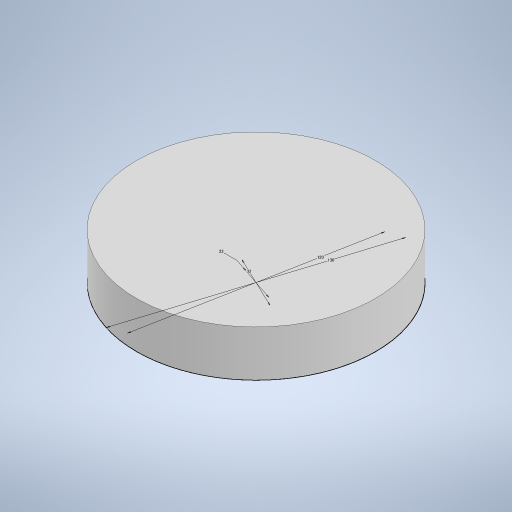
# Autodesk Inventor part: 18-1
Saved by Autodesk Inventor 2023 (Build 270158000, 158)
## iProperties
Created: 2022-11-18
Part Number: 18-1
Material: 一般
Document SubType Name: Modeling
Designer: RM206user
Density: 1 g/cm^3
Appearance: 既定
Author: RM206user
Autodesk Inventor part; units mm, degrees
ref_plane "YZ Plane" through (0, 0, 0) normal (1, 0, 0) x (0, 1, 0)
ref_plane "XZ Plane" through (0, 0, 0) normal (0, 1, 0) x (-1, 0, 0)
ref_plane "XY Plane" through (0, 0, 0) normal (0, 0, 1) x (1, 0, 0)
sketch "スケッチ1" plane through (0, 0, 0) normal (0, 1, 0) x (-1, 0, 0)
  circle A0 centre (0, 0) radius 65
  circle A1 centre (0, 0) radius 60
  circle A2 centre (0, 0) radius 16
  circle A3 centre (0, 0) radius 11
  dimension "d0" = 130
  dimension "d3" = 120
  dimension "d4" = 32
  dimension "d5" = 22
  constraints: 4 centre point, 4 coincident
  measures "d0" diameter of A0
  measures "d3" diameter of A1
  measures "d4" diameter of A2
  measures "d5" diameter of A3
extrude "押し出し1" add sketch "スケッチ1" along normal blind 25 contours A0 | A1 | A2 | A3
extrude "押し出し2" cut sketch "スケッチ1" along normal blind 20 contours A1
extrude "押し出し3" cut sketch "スケッチ1" along normal blind 9 contours A3
